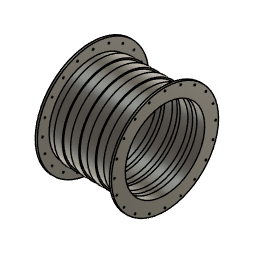
air_turbine_case_eng_model (Autodesk Fusion 360 design; units mm, degrees)
Autodesk Fusion 360 part; units mm, degrees
sketch "Sketch1" plane through (0, 0, 0) normal (0, 1, 0) x (1, 0, 0)
  line L0 (0, 0) -> (179, 0) construction
  line L1 (179, 0) -> (179, -135) construction
  line L2 (179, -135) -> (0, -135) construction
  line L3 (0, -135) -> (0, 0) construction
  line L4 (0, -135) -> (0, -101.42)
  dimension "d1" = 179
  dimension "d2" = 135
  dimension "d3" = 101.42
  constraint horizontal L0
  constraint vertical L1
  constraint horizontal L2
  constraint vertical L3
  constraint coincident L0.start L3.end
  constraint coincident L3 L4.end
  measures "d1" distance of L0.start L0.end
  measures "d2" distance of L0.start L2.end
  measures "d3" distance of L0.start L4.end
sketch "Sketch2" plane through (0, 0, 0) normal (0, 1, 0) x (1, 0, 0)
  line L0 (0, 0) -> (160, 0) construction
  line L1 (179, -135) -> (0, -135) construction
  line L2 (0, -135) -> (0, 0) construction
  line L3 (0, -135) -> (0, -101.42)
  line L4 (80, -98.0476) -> (80, -100.5515)
  line L5 (40, -100.284) -> (40, -102.7879)
  line L6 (120, -95.8113) -> (120, -98.3152)
  line L7 (80, -100.5515) -> (70, -101.1106)
  line L8 (60, -99.1658) -> (70, -101.1106)
  line L9 (60, -99.1658) -> (40, -100.284)
  line L10 (40, -102.7879) -> (30, -103.347)
  line L11 (20, -101.4021) -> (30, -103.347)
  line L12 (160.0645, -96.0752) -> (149.3716, -96.6731)
  line L13 (140, -94.6931) -> (149.3716, -96.6731)
  line L14 (140, -94.6931) -> (120, -95.8113)
  line L15 (120, -98.3152) -> (110, -98.8743)
  line L16 (100, -96.9295) -> (110, -98.8743)
  line L17 (100, -96.9295) -> (80, -98.0476)
  line L18 (0, -101.42) -> (20, -101.4021)
  line L19 (160.0645, -96.0752) -> (179, -96.0752)
  line L20 (179, 0) -> (179, -135)
  line L21 (179, -96.0752) -> (179, -129.65)
  line L22 (179, -129.65) -> (174, -129.65)
  line L23 (0, -135) -> (5, -135)
  line L24 (5, -135) -> (5, -106.42)
  line L25 (174, -129.65) -> (174, -106.42)
  line L26 (5, -106.42) -> (20, -106.42)
  line L27 (20, -106.42) -> (20, -109.42)
  line L28 (20, -109.42) -> (40, -109.42)
  line L29 (40, -109.42) -> (40, -106.42)
  line L30 (40, -106.42) -> (60, -106.42)
  line L31 (60, -106.42) -> (60, -109.42)
  line L32 (60, -109.42) -> (80, -109.42)
  line L33 (80, -109.42) -> (80, -106.42)
  line L34 (80, -106.42) -> (100, -106.42)
  line L35 (100, -106.42) -> (100, -109.42)
  line L36 (100, -109.42) -> (120, -109.42)
  line L37 (120, -109.42) -> (120, -106.42)
  line L38 (120, -106.42) -> (140, -106.42)
  line L39 (140, -106.42) -> (140, -109.42)
  line L40 (140, -109.42) -> (160, -109.42)
  line L41 (160, -109.42) -> (160, -106.42)
  line L42 (160, -106.42) -> (174, -106.42)
  point P0 (179, 0)
  dimension "d4" = 179
  dimension "d5" = 135
  dimension "d6" = 101.42
  dimension "d7" = 129.65
  dimension "d8" = 5
  dimension "d9" = 5
  dimension "d10" = 5
  dimension "d12" = 15
  dimension "d13" = 109.42
  dimension "d14" = 20
  dimension "d15" = 20
  dimension "d16" = 3
  dimension "d17" = 20
  dimension "d18" = 3
  dimension "d19" = 20
  dimension "d20" = 3
  dimension "d21" = 20
  dimension "d22" = 20
  dimension "d23" = 3
  dimension "d24" = 20
  dimension "d25" = 3
  constraint horizontal L0
  constraint horizontal L1
  constraint vertical L2
  constraint coincident L0.start L2.end
  constraint coincident L2 L3.end
  constraint coincident L20 L21.end
  constraint perpendicular L19 L21
  constraint perpendicular L20 L22
  constraint coincident L1 L23.end
  constraint perpendicular L3 L23
  constraint perpendicular L1 L24
  constraint perpendicular L22 L25
  constraint perpendicular L24 L26
  constraint perpendicular L26 L27
  constraint perpendicular L27 L28
  constraint perpendicular L26 L29
  constraint perpendicular L29 L30
  constraint perpendicular L30 L31
  constraint perpendicular L31 L32
  constraint perpendicular L32 L33
  constraint perpendicular L33 L34
  constraint perpendicular L34 L35
  constraint perpendicular L35 L36
  constraint perpendicular L36 L37
  constraint perpendicular L37 L38
  constraint perpendicular L38 L39
  constraint perpendicular L39 L40
  constraint perpendicular L40 L41
  constraint perpendicular L25 L42
  measures "d4" distance of L1.start L1.end
  measures "d5" distance of L1 L0.start
  measures "d6" distance of L0.start L3.end
  measures "d7" distance of L21.end P0
  measures "d8" distance of L21.end L22.end
  measures "d9" distance of L1.end L23.end
  measures "d10" vertical distance of L3.end L24.end
  measures "d12" distance of L24.end L26.end
  measures "d13" vertical distance of L0.start L27.end
  measures "d15" distance of L29.end L30.end
  measures "d16" distance of L30.end L31.end
  measures "d17" distance of L31.end L32.end
  measures "d18" distance of L32.end L33.end
  measures "d19" distance of L33.end L34.end
  measures "d20" distance of L34.end L35.end
  measures "d21" distance of L35.end L36.end
  measures "d22" distance of L37.end L38.end
  measures "d23" distance of L38.end L39.end
  measures "d24" distance of L39.end L40.end
  measures "d25" distance of L40.end L41.end
revolve "Revolve1" add sketch "Sketch2" angle 360 about axis through (0, 0, 0) along (1, 0, 0)
sketch "Sketch3" plane through (0, 0, 0) normal (-1, 0, 0) x (0, -1, 0)
  circle A0 centre (0, 0) radius 135
  circle A1 centre (0, 0) radius 101.42
  line L0 (0, 0) -> (0, 166.4632) construction
  circle A2 centre (0, 122.55) radius 2
  dimension "d27" = 4
  dimension "d28" = 122.55
  constraint coincident A0.centre A1.centre
  constraint vertical L0
  constraint coincident L0 A2.centre
  measures "d27" diameter of A2
  measures "d28" distance of A0.centre A2.centre
extrude "Extrude1" cut sketch "Sketch3" against normal blind 12 contours A2
pattern_circular "C-Pattern1" count 20 over 360 about axis through (1.75, 0, 0) along (1, 0, 0) of "Extrude1"
sketch "Sketch4" plane through (179, 0, 0) normal (1, 0, 0) x (0, 1, 0)
  circle A0 centre (0, 0) radius 96.0752
  circle A1 centre (0, 0) radius 129.65
  line L0 (0, 0) -> (0, 177.3715) construction
  circle A2 centre (0, 122.5) radius 2
  dimension "d33" = 4
  dimension "d34" = 122.5
  constraint coincident A0.centre A1.centre
  constraint vertical L0
  constraint coincident L0 A2.centre
  measures "d33" diameter of A2
  measures "d34" distance of A0.centre A2.centre
extrude "Extrude2" cut sketch "Sketch4" against normal blind 13 contours A2
pattern_circular "C-Pattern2" count 20 over 360 about axis through (1.75, 0, 0) along (1, 0, 0) of "Extrude2"
